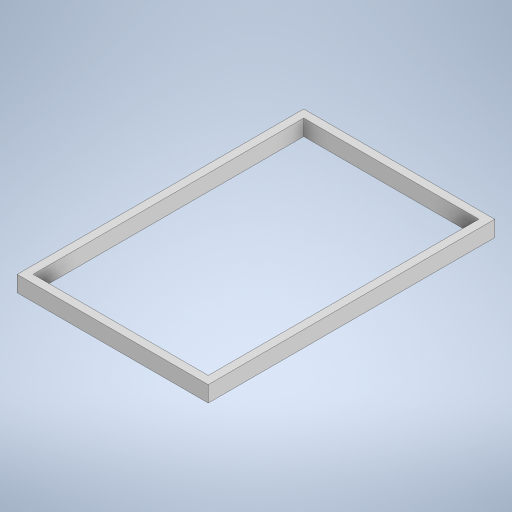
# Autodesk Inventor part: Base stock holder
Saved by Autodesk Inventor 2023 (Build 270158000, 158)
## iProperties
Created: 2022-08-18
Part Number: Base stock holder
Material: Generic
Document SubType Name: Modeling
Designer: rkant
Density: 1 g/cm^3
Appearance: Default
Author: rkant
Autodesk Inventor part; units mm, degrees
ref_plane "YZ Plane" through (0, 0, 0) normal (1, 0, 0) x (0, 1, 0)
ref_plane "XZ Plane" through (0, 0, 0) normal (0, 1, 0) x (-1, 0, 0)
ref_plane "XY Plane" through (0, 0, 0) normal (0, 0, 1) x (1, 0, 0)
sketch "Sketch2" plane through (0, 0, 0) normal (0, 1, 0) x (-1, 0, 0)
  line L0 (304.8, 457.2) -> (-304.8, 457.2)
  line L1 (-304.8, 457.2) -> (-304.8, -457.2)
  line L2 (-304.8, -457.2) -> (304.8, -457.2)
  line L3 (304.8, -457.2) -> (304.8, 457.2)
  point P0 (0, 0)
  point P1 (304.8, 0)
  point P2 (0, 457.2)
  dimension "d4" = 609.6
  dimension "d5" = 914.4
  constraints: 8 end point, 2 midpoint, 2 parallel, 1 horizontal, 1 horizontal alignment, 1 perpendicular, 1 vertical alignment
  measures "d4" distance of L1.end L2.end
  measures "d5" distance of L0.end L1.end
extrude "Extrusion2" add sketch "Sketch2" along normal blind 50.8
sketch "Sketch3" plane through (0, 50.8, 0) normal (0, 1, 0) x (1, 0, 0)
  line L0 (279.4, -431.8) -> (279.4, 431.8)
  line L1 (279.4, 431.8) -> (-279.4, 431.8)
  line L2 (-279.4, 431.8) -> (-279.4, -431.8)
  line L3 (-279.4, -431.8) -> (279.4, -431.8)
  line L4 (279.4, -431.8) -> (-279.4, 431.8) construction
  line L5 (279.4, 431.8) -> (-279.4, -431.8) construction
  line L6 (-279.4, -431.8) -> (-304.8, -431.8)
  line L7 (-304.8, 457.2) -> (-304.8, -457.2) projected
  line L8 (-279.4, -431.8) -> (-279.4, -457.2)
  line L9 (279.4, -431.8) -> (279.4, -457.2)
  line L10 (-304.8, -457.2) -> (304.8, -457.2) projected
  line L11 (279.4, -431.8) -> (304.8, -431.8)
  line L12 (304.8, -457.2) -> (304.8, 457.2) projected
  line L13 (279.4, 431.8) -> (304.8, 431.8)
  line L14 (279.4, 431.8) -> (279.4, 457.2)
  line L15 (-279.4, 431.8) -> (-304.8, 431.8)
  line L16 (-279.4, 431.8) -> (-279.4, 457.2)
  line L17 (304.8, 457.2) -> (-304.8, 457.2) projected
  point P0 (0, 0)
  dimension "d8" = 863.6
  dimension "d9" = 558.8
  constraints: 28 end point, 7 point on line, 4 perpendicular, 3 parallel, 3 vertical, 2 midpoint, 1 horizontal
  measures "d8" distance of L0.start L0.end
  measures "d9" distance of L1.end L0.end
extrude "Extrusion3" cut sketch "Sketch3" against normal blind 50.8 contours L3 L2 L1 L0
body "Solid2"
